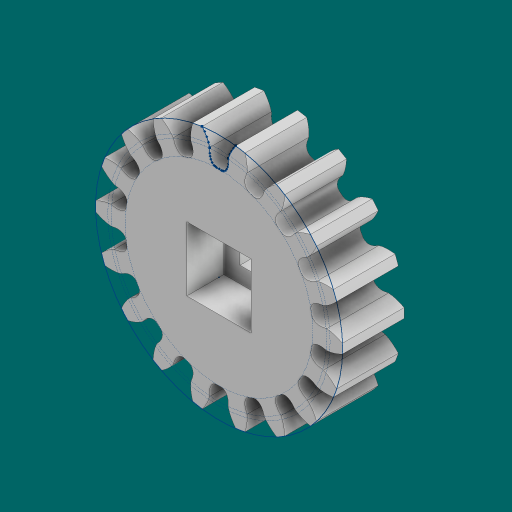
# Autodesk Inventor part: diff_short_gear
Saved by Autodesk Inventor 2023.1 (Build 271208000, 208)
## iProperties
Created: 2022-11-06
Part Number: diff_short_gear
Material: Generic
Document SubType Name: Modeling
Designer: zac-h
Density: 1 g/cm^3
Appearance: Default
Author: zac-h
Autodesk Inventor part; units mm, degrees
ref_plane "YZ Plane" through (0, 0, 0) normal (1, 0, 0) x (0, 1, 0)
ref_plane "XZ Plane" through (0, 0, 0) normal (0, 1, 0) x (-1, 0, 0)
ref_plane "XY Plane" through (0, 0, 0) normal (0, 0, 1) x (1, 0, 0)
sketch "Sketch1" plane through (0, 0, 0) normal (0, 0, 1) x (1, 0, 0)
  spline S0 degree 3 poles (-1.7273, 12.582) (-1.6438, 12.4679) (-1.4768, 12.2397) (-1.2626, 11.8737) (-1.0745, 11.4922) (-0.9995, 11.2194) (-0.962, 11.083) knots 0 0 0 0 0.250092 0.500174 0.750206 1 1 1 1
  spline S1 degree 3 poles (-0.962, 11.083) (-0.9698, 10.9126) (-0.9815, 10.657) (-0.9264, 10.3198) (-0.8448, 10.0768) (-0.7105, 9.8565) (-0.5417, 9.7192) (-0.3826, 9.656) (-0.2126, 9.6346) (0, 9.6483) (0.2126, 9.6346) (0.3826, 9.656) (0.5417, 9.7192) (0.7105, 9.8565) (0.8448, 10.0768) (0.9264, 10.3198) (0.9815, 10.657) (0.9698, 10.9126) (0.962, 11.083) knots 0 0 0 0 0.125027 0.18759 0.250147 0.312625 0.374907 0.406212 0.43741 0.5 0.56259 0.593788 0.625093 0.687375 0.749853 0.81241 0.874973 1 1 1 1
  spline S2 degree 3 poles (0.962, 11.083) (0.9995, 11.2194) (1.0745, 11.4922) (1.2626, 11.8737) (1.4768, 12.2397) (1.6438, 12.4679) (1.7273, 12.582) knots 0 0 0 0 0.249794 0.499826 0.749908 1 1 1 1
  circle A0 centre (0, 0) radius 9.6428 construction
  circle A1 centre (0, 0) radius 11.0659 construction
  circle A2 centre (0, 0) radius 11.43 construction
  circle A3 centre (0, 0) radius 12.7
  point P0 (-1.4829, 12.2358)
  point P1 (-1.2669, 11.8711)
  point P2 (-1.087, 11.4875)
  point P3 (-0.9619, 10.5731)
  point P4 (-0.9197, 10.3214)
  point P5 (-0.8359, 10.0804)
  point P6 (-0.699, 9.8656)
  point P7 (-0.5002, 9.7074)
  point P8 (-0.3812, 9.6612)
  point P9 (-0.2553, 9.6427)
  point P10 (0, 9.6428)
  point P11 (0.2553, 9.6427)
  point P12 (0.3812, 9.6612)
  point P13 (0.5002, 9.7074)
  point P14 (0.699, 9.8656)
  point P15 (0.8359, 10.0804)
  point P16 (0.9197, 10.3214)
  point P17 (0.9619, 10.5731)
  point P18 (1.087, 11.4875)
  point P19 (1.2669, 11.8711)
  point P20 (1.4829, 12.2358)
  constraints: 4 centre point, 2 point on circle, 57 other
extrude "Extrusion1" add sketch "Sketch1" against normal blind 6.35
extrude "Extrusion2" cut sketch "Sketch1" against normal through all contours A3 S2 S1 S0 picked at (0.2047, 11.9455)
pattern_circular "Circular Pattern1" count 18 over 360 about axis through (0, 0, 0) along (0, 0, -1) of "Extrusion2"
sketch "Sketch2" plane through (0, 0, 0) normal (0, 0, 1) x (1, 0, 0)
  line L0 (-1.651, -1.651) -> (1.651, -1.651)
  line L1 (1.651, -1.651) -> (1.651, 1.651)
  line L2 (1.651, 1.651) -> (-1.651, 1.651)
  line L3 (-1.651, 1.651) -> (-1.651, -1.651)
  line L4 (-1.651, -1.651) -> (1.651, 1.651) construction
  line L5 (1.651, -1.651) -> (-1.651, 1.651) construction
  point P0 (0, 0)
  dimension "d7" = 3.302
  dimension "d8" = 3.302
  constraints: 12 end point, 2 midpoint, 2 parallel, 1 horizontal, 1 perpendicular
  measures "d7" distance of L2.end L1.end
  measures "d8" distance of L1.end L0.end
extrude "Extrusion3" cut sketch "Sketch2" against normal through all
sketch "Sketch3" plane through (0, 0, 0) normal (0, 0, 1) x (1, 0, 0)
  line L0 (-3.302, -3.302) -> (3.302, -3.302)
  line L1 (3.302, -3.302) -> (3.302, 3.302)
  line L2 (3.302, 3.302) -> (-3.302, 3.302)
  line L3 (-3.302, 3.302) -> (-3.302, -3.302)
  line L4 (-3.302, -3.302) -> (3.302, 3.302) construction
  line L5 (3.302, -3.302) -> (-3.302, 3.302) construction
  point P0 (0, 0)
  dimension "d11" = 6.604
  dimension "d12" = 6.604
  constraints: 12 end point, 2 midpoint, 2 parallel, 1 horizontal, 1 perpendicular
  measures "d11" distance of L2.end L1.end
  measures "d12" distance of L1.end L0.end
extrude "Extrusion4" cut sketch "Sketch3" against normal blind 3.81
sketch "Sketch4" plane through (0, 0, -6.35) normal (0, 0, -1) x (-1, 0, 0)
  circle A0 centre (0, 0) radius 4.191
  line L0 (1.651, -1.651) -> (-1.651, -1.651) projected
  line L1 (1.651, 1.651) -> (1.651, -1.651) projected
  line L2 (-1.651, 1.651) -> (1.651, 1.651) projected
  line L3 (-1.651, -1.651) -> (-1.651, 1.651) projected
  dimension "d15" = 8.382
  constraints: 1 centre point, 1 coincident
  measures "d15" diameter of A0
extrude "Extrusion5" add sketch "Sketch4" along normal blind 1.27
chamfer "Chamfer1" distance 0.3 angle 45 2 edges at (4.191, 0, -6.35) (4.191, 0, -7.62)
equation "\"d0\" = FaceWidth"
equation "\"Module\" = 1.27"
equation "\"PressureAngle\" = 14.5deg"
equation "\"UnitProfileClearance\" = 0.25"
equation "\"UnitRoundRadius\" = 0.3335"
equation "\"HeadDiameter\" = 25.4"
equation "\"RootDiameter\" = 19.28561"
equation "\"BaseDiameter\" = 22.13186"
equation "\"PitchDiameter\" = 22.86"
equation "\"FaceWidth\" = 6.35"
equation "\"HelixAngle\" = 0"
equation "\"UnitCorrection\" = 0"
equation "\"UnitAddendumModification\" = 0"
equation "\"CircularPitch\" = 3.98982"
equation "\"UnitBacklashShift\" = -0.157241"
equation "\"TotalToolShift\" = -0.1997"
equation "\"IsInternal\" = 0"
body "Solid1"
